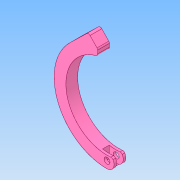
# Autodesk Inventor part: BearingHolder1
Saved by Autodesk Inventor 2017.3 (Build 213256000, 256)
## iProperties
Created: 2019-06-19
Part Number: BearingHolder1
Material: ABS Plastic
Document SubType Name: Modeling
Designer: Derek Wider
Density: 1.06 g/cm^3
Appearance: Pink
Author: Derek Wider
Autodesk Inventor part; units mm, degrees
ref_plane "XZ Plane" through (0, 0, 0) normal (0, 1, 0) x (-1, 0, 0)
ref_plane "XY Plane" through (0, 0, 0) normal (0, 0, 1) x (1, 0, 0)
sketch "Sketch1" plane through (0, 0, 0) normal (0, 0, 1) x (1, 0, 0)
  line L0 (0, 0) -> (4.826, 4.3221)
  line L1 (4.826, 4.3221) -> (10.16, 0)
  line L2 (10.16, 0) -> (11.43, 6.2217)
  line L3 (0, 0) -> (-4.975, 5.229)
  arc A0 (11.43, 6.2217) -> (-4.975, 5.229) centre (5.08, -24.8868) ccw
  circle A1 centre (5.08, -24.8868) radius 25.4 construction
  circle A2 centre (5.08, -24.8868) radius 21.59 construction
  arc A3 (5.08, -47.1118) -> (7.7653, -46.949) centre (5.08, -24.8868) ccw
  circle A4 centre (5.08, -49.6518) radius 1.5875
  line L4 (5.08, -49.6518) -> (5.08, -46.4768) construction
  arc A5 (-14.879, -4.4376) -> (5.08, -53.4618) centre (5.08, -24.8868) ccw
  arc A6 (5.08, -53.4618) -> (7.7653, -46.949) centre (5.08, -49.6518) ccw
  line L5 (0, 0) -> (0, -3.2502)
  line L6 (-4.975, 5.229) -> (-14.879, -4.4376)
  arc A7 (0, -3.2502) -> (5.08, -47.1118) centre (5.08, -24.8868) ccw
  dimension "d40" = 43.18
  dimension "d0" = 31.75
  dimension "d2" = 50.8
  dimension "d3" = 29.21
  dimension "d4" = 30
  dimension "d5" = 10.16
  dimension "d6" = 5.334
  dimension "d42" = 44.45
  dimension "d43" = 3.175
  dimension "d44" = 3.175
  dimension "d47" = 3.81
  constraints: 14 end point, 12 point on circle, 7 centre point, 4 coincident, 2 tangent, 2 vertical, 2 vertical alignment, 1 concentric, 1 horizontal alignment, 1 line through centre, 1 point on line, 2 other
  measures "d0" radius of A0
  measures "d2" diameter of A1
  measures "d3" distance of A1.centre L0.end
  measures "d5" distance of L1.end L0.start
  measures "d6" horizontal distance of L1.end L0.end
  measures "d42" diameter of A3
  measures "d43" diameter of A4
  measures "d44" distance of L4.start L4.end
  measures "d47" radius of A6
extrude "Extrusion1" add sketch "Sketch1" along normal blind 6.35 contours L5 A7 A3 A6 A5 L6 L3
ref_plane "Work Plane1" through (8.89, -49.6518, 0) normal (1, 0, 0) x (0, 1, 0)
sketch "Sketch5" plane through (8.89, -49.6518, 0) normal (1, 0, 0) x (0, 1, 0)
  line L0 (-1.5875, 6.35) -> (1.5875, 6.35) construction
  line L1 (1.5875, 0) -> (-1.5875, 0) construction
  line L2 (-3.556, 1.397) -> (3.556, 1.397)
  line L3 (3.556, 1.397) -> (3.556, 4.953)
  line L4 (3.556, 4.953) -> (-3.556, 4.953)
  line L5 (-3.556, 4.953) -> (-3.556, 1.397)
  line L6 (-3.81, 0) -> (-3.81, 6.35) construction
  point P0 (49.6518, 0)
  point P1 (3.556, 3.175)
  point P2 (-3.81, 3.175)
  point P3 (0, 4.953)
  point P4 (0, 6.35)
  dimension "d48" = 3.556
  dimension "d49" = 7.112
  constraints: 8 end point, 4 midpoint, 2 parallel, 1 horizontal, 1 horizontal alignment, 1 perpendicular, 1 vertical alignment
  measures "d48" distance between parallel lines of L2 L4
  measures "d49" distance of L3.end L4.end
extrude "Extrusion5" cut sketch "Sketch5" against normal blind 7.62
fillet "Fillet2" radius 1.27 5 edges at (7.7653, -46.949, 5.6515) (7.7653, -46.949, 0.6985) (0, -3.2502, 3.175) (0, 0, 3.175) (-4.975, 5.229, 3.175)
body "Solid1"
